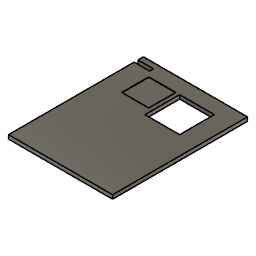
Top_level v55 (Autodesk Fusion 360 archive; units mm, degrees)
design "RF_plate"
Autodesk Fusion 360 part; units mm, degrees
box "BoxPrimitive1" add length 175 width 195 height 5 placed x (0, 1, 0) y (-1, 0, 0) z (0, 0, 1) at (195, 0, 0) makes body 1
cylinder "CylinderPrimitive2" add diameter 50 height 10 placed x (1, 0, 0) y (0, 1, 0) z (0, 0, 1) at (0, 0, 5) separate body makes body 2
move_body "Move1" bodies 2 to x (1, 0, 0) y (0, 1, 0) z (0, 0, 1) at (90, 87.5, -5)
extrude "Extrude1" cut 1 faces at (83.2241, 86.258, 10) along direction (0, 0, -1) blind 80 on bodies 2 bodies 1 2
cylinder "CylinderPrimitive3" add diameter 5 height 5 placed x (1, 0, 0) y (0, 1, 0) z (0, 0, 1) at (0, 0, 5) separate body makes body 3
move_body "Move2" bodies 3 to x (1, 0, 0) y (0, 1, 0) z (0, 0, 1) at (10, 87.5, 0)
extrude "Extrude2" cut 1 faces at (9.4804, 87.9821, 10) along direction (0, 0, -1) blind 5.5 on bodies 3 bodies 1 3
extrude "Extrude3" cut 1 faces at (195, 116.6667, 1.6667) along direction (-1, 0, 0) blind 30 on bodies 1 bodies 1
extrude "Extrude4" cut 1 faces at (165, 116.6667, 1.6667) along direction (-1, 0, 0) blind 30 on bodies 1 bodies 1
extrude "Extrude5" add 1 faces at (9.4804, 87.9821, 4.5) along direction (0, 0, 1) blind 0.5 on bodies 1 bodies 1 2 3
box "BoxPrimitive2" cut length 10 width 5 height -0.5 placed x (0, 1, 0) y (-1, 0, 0) z (0, 0, 1) at (70, 150, 5) bodies 1
cylinder "CylinderPrimitive4" add diameter 72.111 height 5 placed x (1, 0, 0) y (0, 1, 0) z (0, 0, 1) at (90, 90, 0) bodies 1
box "BoxPrimitive3" cut length 35 width 35 height -0.5 placed x (0, -1, 0) y (1, 0, 0) z (0, 0, 1) at (95, 150, 5) bodies 1
box "BoxPrimitive4" cut length 60 width 40 height -5 placed x (0, -1, 0) y (1, 0, 0) z (0, 0, 1) at (84, 100, 5) bodies 1
sketch "Sketch9" plane through (0, 0, 5) normal (0, 0, 1) x (-1, 0, 0)
  line L0 (-84, -40) -> (-84, -100)
  line L1 (-84, -100) -> (-124, -100)
  line L2 (-124, -100) -> (-124, -40)
  line L3 (-124, -40) -> (-84, -40)
  line L4 (-95, -115) -> (-95, -150)
  line L5 (-95, -150) -> (-130, -150)
  line L6 (-130, -150) -> (-130, -115)
  line L7 (-130, -115) -> (-95, -115)
  line L8 (-70, -160) -> (-70, -150)
  line L9 (-70, -150) -> (-65, -150)
  line L10 (-65, -150) -> (-65, -160)
  line L11 (-65, -160) -> (-70, -160)
  line L12 (-135, 0) -> (-135, -175)
  line L13 (-135, -175) -> (0, -175)
  line L14 (0, -175) -> (0, 0)
  line L15 (0, 0) -> (-135, 0)
box "BoxPrimitive5" cut length 5 width 20 height -23 placed x (0, 1, 0) y (-1, 0, 0) z (0, 0, 1) at (20, 163, 5) bodies 1
extrude "Extrude6" add sketch "Sketch9" along normal blind 0.5 separate body contours L8 L9 L10 L11 makes body 4
extrude "Extrude7" cut 1 faces at (68.3333, 153.3333, 5.5) along direction (0, 0, -1) blind 0.5 on bodies 4 bodies 4
extrude "Extrude8" add 1 faces at (66.6667, 153.3333, 4.5) along direction (0, 0, 1) blind 0.5 on bodies 1 bodies 1 4
extrude "Extrude9" add 1 faces at (118.3333, 138.3333, 4.5) along direction (0, 0, 1) blind 0.5 on bodies 1 bodies 1
extrude "Extrude10" add 1 faces at (110.6667, 40, 1.6667) along direction (0, 1, 0) blind 95 on bodies 1 bodies 1
box "BoxPrimitive6" cut length 35 width 35 height -0.5 placed x (0, 1, 0) y (-1, 0, 0) z (0, 0, 1) at (61, 121, 5) bodies 1
box "BoxPrimitive7" cut length 45 width 45 height -50 placed x (0, 1, 0) y (-1, 0, 0) z (0, 0, 1) at (111, 111, 5) bodies 1

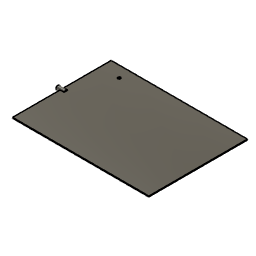
design "Antenna"
Autodesk Fusion 360 part; units mm, degrees
box "BoxPrimitive1" add length 123 width 170 height 1 placed x (0, -1, 0) y (1, 0, 0) z (0, 0, 1) at (0, 0, 0) makes body 1
cylinder "CylinderPrimitive1" add diameter 5 height 10 placed x (0, 0, -1) y (0, 1, 0) z (1, 0, 0) at (0, 10, 10) separate body makes body 2
move_body "Move1" bodies 2 to x (1, 0, 0) y (0, 1, 0) z (0, 0, 1) at (0, -10, -10)
move_body "Move2" bodies 2 to x (1, 0, 0) y (0, 1, 0) z (0, 0, 1) at (0, -61.5, 0)
move_body "Move3" bodies 2 to x (1, 0, 0) y (0, 1, 0) z (0, 0, 1) at (-5, 0, 0)
combine "Combine1" operation add target body 1 tool bodies 2
cylinder "CylinderPrimitive2" cut diameter 3.5 height -1 placed x (1, 0, 0) y (0, 1, 0) z (0, 0, 1) at (24, -14, 1) bodies 1
